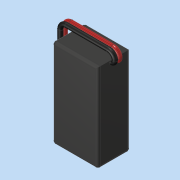
# Autodesk Inventor part: ElectronicsBatteryNoConnector
Saved by Autodesk Inventor 2017 (Build 210142000, 142)
## iProperties
Created: 2018-02-14
Part Number: ElectronicsBatteryNoConnector
Material: PBT Plastic
Document SubType Name: Modeling
Designer: Derek Wider
Density: 2.07838 g/cm^3
Appearance: Smooth - Black
Mass: 136.078 g
Surface Area: 118.78 cm^2
Volume: 65.4728 cm^3
Author: Derek Wider
Autodesk Inventor part; units mm, degrees
ref_plane "YZ Plane" through (0, 0, 0) normal (1, 0, 0) x (0, 1, 0)
ref_plane "XZ Plane" through (0, 0, 0) normal (0, 1, 0) x (-1, 0, 0)
ref_plane "XY Plane" through (0, 0, 0) normal (0, 0, 1) x (1, 0, 0)
sketch "Sketch1" plane through (0, 0, 0) normal (0, 1, 0) x (-1, 0, 0)
  line L0 (0, 0) -> (36, 0)
  line L1 (36, 0) -> (36, -25.5)
  line L2 (36, -25.5) -> (0, -25.5)
  line L3 (0, -25.5) -> (0, 0)
  dimension "d0" = 36
  dimension "d1" = 25.5
  constraints: 8 end point, 2 parallel, 1 horizontal, 1 perpendicular
  measures "d0" distance of L1.end L2.end
  measures "d1" distance of L0.end L1.end
extrude "Extrusion1" add sketch "Sketch1" along normal blind 70
sketch "Sketch2" plane through (0, 0, 0) normal (1, 0, 0) x (0, 0, -1)
  circle A0 centre (10.8862, 68.25) radius 1.75
  circle A1 centre (14.3862, 68.25) radius 1.75
  line L0 (0, 70) -> (25.5, 70) projected
  line L1 (10.8862, 68.25) -> (-0.2275, 68.25) construction
  line L2 (14.3862, 68.25) -> (25.5, 68.25) construction
  line L3 (25.5, 0) -> (25.5, 70) construction
  point P0 (0, 0)
  dimension "d4" = 3.5
  constraints: 4 end point, 3 tangent, 2 centre point, 2 horizontal, 1 collinear, 1 equal radius, 1 point on line
  measures "d4" diameter of A0
sketch "Sketch4" plane through (-36, 0, 0) normal (0, 0, 1) x (1, 0, 0)
  line L0 (0, 70) -> (36, 70) construction
  line L1 (36, 0) -> (36, 70) construction
  arc A0 (36, 68.25) -> (38.5, 70.75) centre (36, 70.75) ccw
  line L2 (33.5, 75.75) -> (0.5, 75.75)
  arc A1 (38.5, 70.75) -> (33.5, 75.75) centre (33.5, 70.75) ccw
  line L3 (-4.5, 55.75) -> (-4.5, 70.75)
  arc A2 (0.5, 75.75) -> (-4.5, 70.75) centre (0.5, 70.75) ccw
  line L4 (0, 0) -> (0, 70) projected
  dimension "d6" = 2.5
  dimension "d7" = 5
  dimension "d8" = 1.75
  dimension "d9" = 4.5
  dimension "d10" = 15
  constraints: 6 point on circle, 4 end point, 4 tangent, 3 centre point, 1 equal radius, 1 horizontal, 1 horizontal alignment, 1 point on line, 1 vertical, 1 vertical alignment
  measures "d6" radius of A0
  measures "d7" radius of A1
  measures "d8" distance of A0.start L0.end
  measures "d9" distance between parallel lines of L4 L3
  measures "d10" distance of L3.start L3.end
sweep "Sweep1" add profiles "Sketch2" path "Sketch4" path curves A0 A1 L2 A2 L3 contours A0 | A1
sketch "Sketch6" plane through (-40.5, 55.75, -10.8862) normal (0, -1, 0) x (1, 0, 0)
  circle A0 centre (0, -3.5) radius 1.75 projected
  circle A1 centre (0, 0) radius 1.75 projected
  point P0 (40.5, 10.8862)
  point P1 (0, -1.75)
  point P2 (0, -1.75)
  constraints: 2 vertical alignment
sketch "Sketch5" plane through (-36, 0, -25.5) normal (-1, 0, 0) x (0, 0, 1)
  line L0 (12.8638, 55.75) -> (16.3638, 55.75) construction
  line L1 (9.3638, 70.75) -> (12.8638, 70.75) construction
  line L2 (12.8638, 70.75) -> (12.8638, 55.75) construction
  line L3 (9.3638, 55.75) -> (12.8638, 55.75) construction
  line L4 (12.8638, 55.75) -> (12.8638, 38.2887) construction
  line L5 (14.6138, 55.75) -> (14.6138, 48.25) construction
  line L6 (14.6138, 48.25) -> (16.8008, 48.25) construction
  line L7 (16.8008, 48.25) -> (16.8008, 40.75) construction
  spline S0 degree 3 poles (14.6138, 55.75) (14.6138, 48.25) (16.8008, 48.25) (16.8008, 40.75) knots 1 1 1 1 2 2 2 2
  line L8 (16.8008, 40.75) -> (16.8008, 38.75)
  line L9 (11.1138, 55.75) -> (11.1138, 48.25) construction
  line L10 (11.1138, 48.25) -> (8.9268, 48.25) construction
  line L11 (8.9268, 48.25) -> (8.9268, 40.75) construction
  spline S1 degree 3 poles (11.1138, 55.75) (11.1138, 48.25) (8.9268, 48.25) (8.9268, 40.75) knots 1 1 1 1 2 2 2 2
  line L12 (8.9268, 40.75) -> (8.9268, 38.75)
  point P0 (25.5, 0)
  dimension "d13" = 3.937
  dimension "d14" = 15
  dimension "d15" = 2
  constraints: 6 end point, 5 symmetric about line, 3 vertical, 1 horizontal, 1 midpoint, 1 parallel, 1 point on line, 6 other
  measures "d13" distance from line of L4 L7.end
  measures "d14" vertical distance of L5.start L7.end
  measures "d15" distance of L7.end L8.end
sweep "Sweep2" add profiles "Sketch6" path "Sketch5" path curves S0 L8 contours A1
sweep "Sweep3" add profiles "Sketch6" path "Sketch5" path curves S1 L12 contours A0
fillet "Fillet1" radius 2 11 edges at (0, 35, 0) (0, 35, -25.5) (0, 0, -12.75) (-18, 0, -25.5) (-18, 0, 0) (-18, 70, -25.5) (-36, 35, -25.5) (-36, 0, -12.75) (-36, 35, 0) (-18, 70, 0) (-36, 70, -12.75)
sketch "Sketch7" plane through (-2, 2, -25.5) normal (0, 0, -1) x (-1, 0, 0)
  line L0 (28.8742, 63.6567) -> (28.8742, 4.0173) construction
  line L1 (28.8742, 4.0173) -> (3.4367, 4.0173) construction
  line L2 (3.4367, 4.0173) -> (3.4367, 63.6567) construction
  line L3 (3.4367, 63.6567) -> (28.8742, 63.6567) construction
  constraints: 2 other
body "Solid1"
